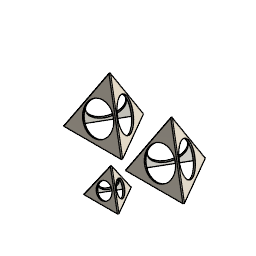
Oct25_Tripod (Autodesk Fusion 360 design; units mm, degrees)
part number: 2025-10-25-14-16-04-339
part number: 2025-10-25-14-21-02-977
part number: 2025-10-25-14-38-52-078
Autodesk Fusion 360 part; units mm, degrees
sketch "Sketch1" plane through (0, 0, 0) normal (0, 0, 1) x (1, 0, 0) in component "Painter's Tripod"
  line L0 (0, 0) -> (50, 86.6025)
  line L1 (50, 86.6025) -> (100, 0)
  line L2 (100, 0) -> (0, 0)
  dimension "d1" = 100
  constraint coincident L0.start L2.end
  constraint horizontal L2
  constraint equal L0 L1
  constraint equal L0 L2
  measures "d1" distance of L0.start L0.end
ref_plane "WorkPlane1" through (0, 0, 90) normal (0, 0, 1) x (1, 0, 0) in component "Painter's Tripod"
sketch "Sketch2" plane through (0, 0, 90) normal (0, 0, 1) x (1, 0, 0) in component "Painter's Tripod"
  line L0 (0, 0) -> (50, 86.6025)
  line L1 (50, 86.6025) -> (100, 0)
  line L2 (100, 0) -> (0, 0)
  line L3 (50, 86.6025) -> (50, 0) construction
  line L4 (0, 0) -> (75, 43.3013) construction
  point P0 (50, 28.8675)
  constraint coincident L0.end L1.start
  constraint midpoint L2 L3.end
  constraint coincident L0.start L2.end
  constraint midpoint L1 L4.end
  constraint coincident L4 P0
  constraint coincident L3 P0
loft "Loft1" add profiles "Sketch1" section 1 section 2 point at (50, 28.8675, 90) makes body 1 in component "Painter's Tripod"
shell "Shell1" thickness 2.5 removed faces 1 at (50, 28.8675, 0) on bodies 1 in component "Painter's Tripod"
sketch "Sketch3" plane through (0, 0, 0) normal (0, -0.952217, 0.305424) x (1, 0, 0) in component "Painter's Tripod"
  line L0 (0, 0) -> (100, 0)
  line L1 (100, 0) -> (50, 94.5163)
  line L2 (50, 94.5163) -> (0, 0)
  line L3 (0, 0) -> (50, 94.5163)
  line L4 (100, 0) -> (50, 94.5163)
  line L5 (100, 0) -> (0, 0)
  line L6 (50, 94.5163) -> (50, 0) construction
  line L7 (0, 0) -> (75, 47.2582) construction
  circle A0 centre (50, 31.5054) radius 25
  dimension "d4" = 50
  constraint coincident L1.end L2.start
  constraint midpoint L0 L6.end
  constraint coincident L0.start L2.end
  constraint midpoint L4 L7.end
  constraint coincident L6 A0.centre
  constraint coincident L7 A0.centre
  measures "d4" diameter of A0
extrude "Extrude1" cut sketch "Sketch3" against normal up to surface (2.5 mm away) contours A0 bodies 1 in component "Painter's Tripod"
pattern_circular "C-Pattern1" count 3 over 360 about axis through (50, 28.8675, 125) along (0, 0, -1) of "Extrude1" in component "Painter's Tripod"
fillet "Fillet1" radius 1 3 edges at (75, 14.4338, 45) (50, 57.735, 45) (25, 14.4338, 45) on bodies 1 in component "Painter's Tripod"
sketch "Sketch1 (2)" plane through (0, 0, 0) normal (0, 0, 1) x (1, 0, 0) in component "Painter's Tripod (1)"
  line L0 (0, 0) -> (30, 51.9615)
  line L1 (30, 51.9615) -> (60, 0)
  line L2 (60, 0) -> (0, 0)
  dimension "d1_1" = 60
  constraint coincident L0.start L2.end
  constraint horizontal L2
  constraint equal L0 L1
  constraint equal L0 L2
  measures "d1_1" distance of L0.start L0.end
ref_plane "WorkPlane1" through (0, 0, 50) normal (0, 0, 1) x (1, 0, 0) in component "Painter's Tripod (1)"
sketch "Sketch2 (2)" plane through (0, 0, 50) normal (0, 0, 1) x (1, 0, 0) in component "Painter's Tripod (1)"
  line L0 (0, 0) -> (30, 51.9615)
  line L1 (30, 51.9615) -> (60, 0)
  line L2 (60, 0) -> (0, 0)
  line L3 (30, 51.9615) -> (30, 0) construction
  line L4 (0, 0) -> (45, 25.9808) construction
  point P0 (30, 17.3205)
  constraint coincident L0.end L1.start
  constraint midpoint L2 L3.end
  constraint coincident L0.start L2.end
  constraint midpoint L1 L4.end
  constraint coincident L4 P0
  constraint coincident L3 P0
loft "Loft1'" add profiles "Sketch1 (2)" section 1 section 2 point at (30, 17.3205, 50) separate body makes body 2 in component "Painter's Tripod (1)"
shell "Shell1'" thickness 2.5 removed faces 1 at (30, 17.3205, 0) on bodies 2 in component "Painter's Tripod (1)"
sketch "Sketch3 (2)" plane through (0, 0, 0) normal (0, -0.944911, 0.327327) x (1, 0, 0) in component "Painter's Tripod (1)"
  line L0 (0, 0) -> (60, 0)
  line L1 (60, 0) -> (30, 52.915)
  line L2 (30, 52.915) -> (0, 0)
  line L3 (0, 0) -> (30, 52.915)
  line L4 (60, 0) -> (30, 52.915)
  line L5 (60, 0) -> (0, 0)
  line L6 (30, 52.915) -> (30, 0) construction
  line L7 (0, 0) -> (45, 26.4575) construction
  circle A0 centre (30, 17.6383) radius 12.5
  dimension "d4_1" = 25
  constraint coincident L1.end L2.start
  constraint midpoint L0 L6.end
  constraint coincident L0.start L2.end
  constraint midpoint L4 L7.end
  constraint coincident L6 A0.centre
  constraint coincident L7 A0.centre
  measures "d4_1" diameter of A0
extrude "Extrude1'" cut sketch "Sketch3 (2)" against normal up to surface (2.5 mm away) contours A0 bodies 2 in component "Painter's Tripod (1)"
pattern_circular "C-Pattern1'" count 3 over 360 about axis through (30, 17.3205, 75) along (0, 0, -1) of "Extrude1'" in component "Painter's Tripod (1)"
fillet "Fillet1'" radius 1 3 edges at (45, 8.6603, 25) (30, 34.641, 25) (15, 8.6603, 25) on bodies 2 in component "Painter's Tripod (1)"
component "Painter's Tripod" placed x (1, 0, 0) y (0, 1, 0) z (0, 0, 1) at (0, 0, 0)
component "Painter's Tripod (1)" placed x (1, 0, 0) y (0, 1, 0) z (0, 0, 1) at (0, 0, 0)
component "Painter's Tripod" placed x (1, 0, 0) y (0, 1, 0) z (0, 0, 1) at (-113.872, 10, 2.5895)
